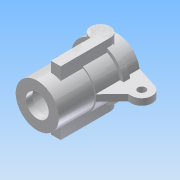
# Autodesk Inventor part: Front Axle Body
Saved by Autodesk Inventor 2014 (Build 180170000, 170)
## iProperties
Created: 2011-09-22
Part Number: Front Axle Body
Document SubType Name: Modeling
Designer: dgitz
Density: 1 g/cm^3
Material: Generic
Appearance: Polished Brushed
Author: dgitz
Autodesk Inventor part; units mm, degrees
ref_plane "YZ Plane" through (0, 0, 0) normal (1, 0, 0) x (0, 1, 0)
sketch "Sketch2" plane through (0, 0, 0) normal (0, 0, 1) x (1, 0, 0)
  circle A0 centre (0, 0) radius 8.382
  dimension "d0" = 16.764
  constraints: 1 centre point, 1 coincident
  measures "d0" diameter of A0
extrude "Extrusion1" add sketch "Sketch2" along normal blind 13.97
sketch "Sketch3" plane through (0, 0, 0) normal (0, 0, -1) x (-1, 0, 0)
  circle A0 centre (0, 0) radius 8.382 projected
  circle A1 centre (0, 0) radius 8.89
  dimension "d3" = 17.78
  constraints: 1 centre point, 1 coincident
  measures "d3" diameter of A1
extrude "Extrusion2" add sketch "Sketch3" along normal blind 17.018 contours A0 | A1
ref_plane "Work Plane1" through (0, 0, -9.398) normal (0, 0, 1) x (1, 0, 0)
sketch "Sketch4" plane through (0, 0, -9.398) normal (0, 0, 1) x (1, 0, 0)
  circle A0 centre (0, 0) radius 8.89
  circle A1 centre (0, 0) radius 10.287
  circle A2 centre (0, 0) radius 8.89 projected
  dimension "d7" = 20.574
  constraints: 2 centre point, 2 coincident, 1 concentric
  measures "d7" diameter of A1
extrude "Extrusion3" add sketch "Sketch4" against normal blind 2.54
sketch "Sketch9" plane through (0, 0, -17.018) normal (0, 0, -1) x (-1, 0, 0)
  circle A0 centre (0, 0) radius 8.89 projected
  circle A1 centre (0, 0) radius 6.985
  dimension "d40" = 13.97
  constraints: 1 centre point, 1 coincident
  measures "d40" diameter of A1
extrude "Extrusion7" cut sketch "Sketch9" against normal blind 28.448 contours A1
sketch "Sketch10" plane through (0, 0, 13.97) normal (0, 0, 1) x (1, 0, 0)
  circle A0 centre (0, 0) radius 8.382 projected
  circle A1 centre (0, 0) radius 4.445
  dimension "d43" = 8.89
  constraints: 1 centre point, 1 coincident
  measures "d43" diameter of A1
extrude "Extrusion8" cut sketch "Sketch10" against normal up to surface (2.54 mm away) contours A1
sketch "Sketch12" plane through (0, 0, 0) normal (0, 1, 0) x (-1, 0, 0)
  line L0 (8.89, -17.018) -> (-8.89, -17.018) projected
  line L1 (-13.7704, -25.0461) -> (-13.7704, -36.5125) construction
  circle A0 centre (-16.256, -10.414) radius 1.524
  arc A1 (-16.256, -6.35) -> (-17.4864, -14.2873) centre (-16.256, -10.414) ccw
  line L2 (-16.256, -6.35) -> (-14.965, -6.35)
  line L3 (-14.965, -6.35) -> (-8.89, 0)
  line L4 (-8.89, 0) -> (-8.89, -9.398) projected
  line L5 (-8.89, -17.018) -> (-17.4864, -14.2873)
  line L6 (-8.89, 0) -> (-8.89, -17.018)
  point P0 (0, 0)
  dimension "d54" = 3.048
  dimension "d55" = 8.128
  dimension "d56" = 6.604
  dimension "d57" = 16.256
  constraints: 10 end point, 2 centre point, 2 perpendicular, 2 point on circle, 2 tangent, 1 coincident, 1 collinear
  measures "d54" diameter of A0
  measures "d55" diameter of A1
  measures "d56" distance from line of A0.centre L0
  measures "d57" horizontal distance of A0.centre point (0, 0)
extrude "Extrusion9" add sketch "Sketch12" along normal mid plane 2.54
sketch "Sketch14" plane through (8.89, -1.27, -9.398) normal (-1, 0, 0) x (0, 0, 1)
  line L0 (0, 0) -> (0, 1.27) projected
  line L1 (0, 0) -> (9.398, 0) projected
  line L2 (9.398, 1.27) -> (9.398, 0) projected
  line L3 (9.398, 1.27) -> (0, 1.27) projected
  line L4 (-7.62, 2.54) -> (9.398, 2.54)
  line L5 (9.398, 2.54) -> (9.398, 0)
  line L6 (9.398, 0) -> (-7.62, 0)
  line L7 (-7.62, 0) -> (-7.62, 2.54)
  constraints: 8 end point, 2 parallel, 1 coincident, 1 horizontal, 1 perpendicular
extrude "Extrusion11" add sketch "Sketch14" along normal up to next contours L6 L7 L4 L5 L3 L0
sketch "Sketch15" plane through (0, 0, -17.018) normal (0, 0, -1) x (-1, 0, 0)
  arc A0 (6.8686, 1.27) -> (-6.8686, 1.27) centre (0, 0) ccw projected
  circle A1 centre (0, 0) radius 6.985
  constraints: 1 centre point, 1 coincident, 1 concentric
extrude "Extrusion12" cut sketch "Sketch15" against normal up to surface (28.448 mm away)
ref_plane "Work Plane8" through (0, 12.4206, 0) normal (0, 1, 0) x (-1, 0, 0)
sketch "Sketch16" plane through (0, 12.4206, 0) normal (0, 1, 0) x (-1, 0, 0)
  arc A0 (-3.7707, -10.668) -> (0.0393, -6.858) centre (0.0393, -10.668) ccw
  line L0 (-10.2083, -9.398) -> (10.287, -9.398) projected
  line L1 (10.287, -11.938) -> (-10.2083, -11.938) projected
  line L2 (-10.2083, -9.398) -> (10.287, -11.938) construction
  line L3 (-3.7707, -10.668) -> (-3.7707, 8.636)
  line L4 (-3.7707, 8.636) -> (0.0393, 8.636)
  line L5 (0.0393, 8.636) -> (0.0393, -6.858)
  line L6 (-8.382, 13.97) -> (8.382, 13.97) projected
  point P0 (0, 0)
  dimension "d63" = 7.62
  dimension "d65" = 3.81
  dimension "d66" = 5.334
  constraints: 8 end point, 2 perpendicular, 2 point on circle, 1 centre point, 1 coincident, 1 midpoint, 1 parallel, 1 tangent
  measures "d63" diameter of A0
  measures "d65" distance of L3.end L4.end
  measures "d66" distance between parallel lines of L4 L6
extrude "Extrusion13" add sketch "Sketch16" against normal up to next
mirror "Mirror2" about plane through (0, 0, 0) normal (0, 1, 0) of "Extrusion13"
body "Solid1"
